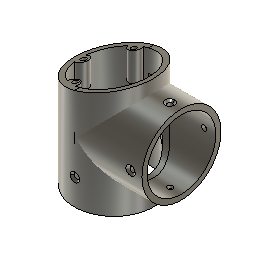
ur5_02_Nema17_Joint (Autodesk Fusion 360 design; units mm, degrees)
part number: 2025-04-09-17-27-22-625
Autodesk Fusion 360 part; units mm, degrees
sketch "Sketch1" plane through (0, 0, 0) normal (0, 0, 1) x (1, 0, 0)
  circle A0 centre (0, 0) radius 38.1
  circle A1 centre (0, 0) radius 33.1
  circle A2 centre (-31, -0.0352) radius 6
  circle A3 centre (-9.8551, -30.4447) radius 6
  circle A4 centre (-9.922, 30.4229) radius 6
  circle A5 centre (-29.55, 0) radius 2.5
  circle A6 centre (-9.1314, -28.1037) radius 2.5
  circle A7 centre (23.9064, -17.369) radius 2.5
  circle A8 centre (23.9064, 17.369) radius 2.5
  circle A9 centre (-9.1314, 28.1037) radius 2.5
  dimension "d1" = 76.2
  dimension "d2" = 5
  dimension "d20" = 12
  dimension "d52" = 5
  dimension "d53" = 1.45
  dimension "d55" = 360
  constraint coincident A0.centre A1.centre
  measures "d1" diameter of A0
  measures "d2" distance of A0 A1
  measures "d20" diameter of A2
  measures "d52" diameter of A5
  measures "d53" horizontal distance of A2.centre A5.centre
extrude "Extrude1" add sketch "Sketch1" along normal blind 117.4 from surface at 35 contours A0 | A1 A4 | A1 A3 | A1 A2 picked at (-10.757, 32.9832) picked at (-10.6845, -33.0067) picked at (-34.3621, -0.039) makes body 1
ref_plane "WorkPlane1" through (85, 0, 0) normal (1, 0, 0) x (0, 1, 0)
sketch "Sketch2" plane through (85, 0, 0) normal (1, 0, 0) x (0, 1, 0)
  circle A0 centre (0, 92.4) radius 38.1
  dimension "d6" = 76.2
  measures "d6" diameter of A0
sketch "Sketch3" plane through (85, 0, 0) normal (1, 0, 0) x (0, 1, 0)
  circle A0 centre (0, 92.4) radius 33.1
  circle A1 centre (0, 92.4) radius 38.1
  dimension "d7" = 5
  measures "d7" distance of A0 A1
extrude "Extrude2" add sketch "Sketch3" against normal blind 65 from surface at -20 separate body makes body 2
extrude "Extrude3" cut sketch "Sketch3" against normal blind 85 contours A0 bodies 1
extrude "Extrude4" cut sketch "Sketch1" along normal blind 160 contours A1 A2 A3 A4 | A1 A4 | A1 A3 | A1 A2 | A5 | A6 | A7 | A8 | A9 picked at (-6.6857, 31.3751) picked at (-6.6392, -31.3856) picked at (-32.1416, -3.3207) bodies 2
ref_plane "WorkPlane2" through (0, -90, 0) normal (0, 1, 0) x (0, 0, 1)
sketch "Sketch4" plane through (0, -90, 0) normal (0, 1, 0) x (1, 0, 0)
  line L0 (-38.1, -152.4) -> (-38.1, -122.4)
  line L1 (-38.1, -152.4) -> (38.1, -152.4)
  line L2 (38.1, -152.4) -> (38.1, -142.4)
  line L3 (38.1, -142.4) -> (-38.1, -122.4)
  dimension "d15" = 30
  dimension "d16" = 76.2
  dimension "d17" = 10
  constraint vertical L0
  constraint perpendicular L0 L1
  constraint perpendicular L1 L2
  measures "d15" distance of L0.start L0.end
  measures "d16" distance of L0.start L1.end
  measures "d17" distance of L1.end L2.end
extrude "Extrude5" cut sketch "Sketch4" along normal blind 150 bodies 1
extrude "Extrude6" add sketch "Sketch1" along normal blind 35 from surface at 102.4 contours A1 A4 | A1 A3 | A1 A2 picked at (-6.6857, 31.3751) picked at (-6.6392, -31.3856) picked at (-32.1416, -3.3207) bodies 1
sketch "Sketch5" plane through (0, -90, 0) normal (0, 1, 0) x (1, 0, 0)
  line L0 (0, -132.4) -> (-38.1, -122.4)
  line L1 (-38.1, -122.4) -> (-38.1, -145)
  line L2 (-38.1, -145) -> (0, -145)
  line L3 (0, -145) -> (0, -132.4)
  constraint vertical L1
  constraint perpendicular L1 L2
  constraint perpendicular L2 L3
extrude "Extrude7" cut sketch "Sketch5" along normal blind 170 bodies 1
sketch "Sketch9" plane through (0, 0, 0) normal (0, 1, 0) x (1, 0, 0)
  circle A0 centre (0, -60) radius 2.5
  line L0 (-38.1, -35) -> (38.1, -35)
  dimension "d56" = 5
  dimension "d57" = 25
  measures "d56" diameter of A0
  measures "d57" distance of A0.centre L0
extrude "Extrude12" cut sketch "Sketch9" along normal mid plane 120 bodies 1
sketch "Sketch10" plane through (0, 0, 0) normal (1, 0, 0) x (0, 0, -1)
  circle A0 centre (-60, 0) radius 2.5
  line L0 (-35, 38.1) -> (-35, -38.1)
  dimension "d60" = 5
  dimension "d61" = 25
  measures "d60" diameter of A0
  measures "d61" distance of A0.centre L0
extrude "Extrude13" cut sketch "Sketch10" against normal blind 60 bodies 1
chamfer "Chamfer1" distance 2 angle 45 4 edges at (2.5, -38.0179, 60) (2.5, 38.0179, 60) (-38.0179, 2.5, 60) (2.5, 38.0179, 60) on bodies 1
sketch "Sketch11" plane through (0, 0, 0) normal (0, 1, 0) x (1, 0, 0)
  line L0 (85, -130) -> (85, -55)
  circle A0 centre (54, -92.5) radius 2.5
  line L1 (65, -130) -> (65, -55)
  dimension "d65" = 5
  dimension "d74" = 11
  constraint vertical L0
  constraint vertical L1
  measures "d65" diameter of A0
  measures "d74" distance of A0.centre L1
extrude "Extrude14" cut sketch "Sketch11" along normal blind 60 bodies 2
pattern_circular "C-Pattern1" count 4 over 360 about axis through (65, 0, 92.4) along (-1, 0, 0) of "Extrude14"
chamfer "Chamfer2" distance 2 angle 45 4 edges at (54, 2.6, 54.3888) (54, -38.0112, 89.8) (54, -2.6, 130.4112) (54, 38.0112, 95) on bodies 2
equation "d74 = 15 mm - 4 mm"
